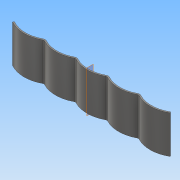
# Autodesk Inventor part: Selection_Selector Sheet
Saved by Autodesk Inventor 2018.1 (Build 221171000, 171)
## iProperties
Created: 2019-02-07
Part Number: Selection_Selector Sheet
Material: Steel, Mild
Document SubType Name: Modeling
Designer: James
Density: 7.85 g/cm^3
Appearance: Semi-Polished
Mass: 244.532 g
Surface Area: 324.289 cm^2
Volume: 31.1506 cm^3
Author: James
Autodesk Inventor part; units mm, degrees
ref_plane "YZ Plane" through (0, 0, 0) normal (1, 0, 0) x (0, 1, 0)
ref_plane "XZ Plane" through (0, 0, 0) normal (0, 1, 0) x (-1, 0, 0)
ref_plane "XY Plane" through (0, 0, 0) normal (0, 0, 1) x (1, 0, 0)
derived "Selection_Skeleton.ipt"
ref_plane "Ground" through (0, 0, 0) normal (0, 1, 0) x (-1, 0, 0)
ref_plane "LHS inner" through (0, 0, 0) normal (1, 0, 0) x (0, 1, 0)
ref_plane "RHS inner" through (300, 0, 0) normal (1, 0, 0) x (0, 1, 0)
ref_plane "Lane 1" through (50, 0, 0) normal (1, 0, 0) x (0, 1, 0)
ref_plane "Lane 2" through (100, 0, 0) normal (1, 0, 0) x (0, 1, 0)
ref_plane "Lane 3" through (150, 0, 0) normal (1, 0, 0) x (0, 1, 0)
ref_plane "Lane 4" through (200, 0, 0) normal (1, 0, 0) x (0, 1, 0)
ref_plane "Lane 5" through (250, 0, 0) normal (1, 0, 0) x (0, 1, 0)
ref_plane "Back" through (0, 0, 0) normal (0, 0, 1) x (1, 0, 0)
sketch "Sketch1" plane through (0, 0, 0) normal (0, 0, 1) x (1, 0, 0)
  line L0 (0, 60) -> (0, -10) projected
  line L1 (300, 60) -> (300, -10) projected
  line L2 (250, 60) -> (250, -10) projected
  line L3 (200, 60) -> (200, -10) projected
  line L4 (150, 60) -> (150, -10) projected
  line L5 (100, 60) -> (100, -10) projected
  line L6 (50, 60) -> (50, -10) projected
  line L7 (-15, 0) -> (90, 0) projected
  arc A0 (25, 9.0244) -> (75, 9.0244) centre (50, 50) ccw
  arc A1 (25, 6.6987) -> (75, 6.6987) centre (50, 50) ccw
  line L8 (25, 9.0244) -> (25, 6.6987)
  line L9 (75, 9.0244) -> (75, 6.6987)
  point P0 (0, 0)
  dimension "d2" = 2
  dimension "d3" = 50
  dimension "d4" = 25
  dimension "d5" = 25
  dimension "d7" = 50
  dimension "d8" = 50
  constraints: 4 end point, 4 point on circle, 2 centre point, 2 vertical alignment, 1 coincident, 1 parallel, 1 point on line, 1 vertical
  measures "d2" radial gap between concentric circles of A0 A1
  measures "d3" distance between parallel lines of L5 L6
  measures "d4" distance from line of L9.start L6
  measures "d5" distance from line of L6 L8.start
  measures "d7" horizontal distance of point (0, 0) A0.centre
  measures "d8" radius of A1
extrude "Extrusion1" add sketch "Sketch1" along normal blind 60
pattern_linear "Rectangular Pattern1" count 5 spacing 50 along (1, 0, 0) of "Extrusion1"
fillet "Fillet1" radius 3 4 edges at (75, 6.6987, 30) (125, 6.6987, 30) (175, 6.6987, 30) (225, 6.6987, 30)
fillet "Fillet2" radius 5 4 edges at (75, 9.0244, 30) (125, 9.0244, 30) (175, 9.0244, 30) (225, 9.0244, 30)
ref_plane "Mid Plane" through (150, 6.6987, 0) normal (-1, 0, 0) x (0, 0, 1)
sketch "Sketch2" plane through (0, 0, 60) normal (0, 0, 1) x (1, 0, 0)
  arc A0 (25, 9.0244) -> (72.6415, 7.6755) centre (50, 50) ccw projected
  arc A1 (25, 6.6987) -> (73.5849, 5.912) centre (50, 50) ccw projected
  line L0 (25, 6.6987) -> (26, 8.4308)
  line L1 (26, 8.4308) -> (50, 50) construction
  line L2 (25, 9.0244) -> (25, 6.6987) projected
  line L3 (25, 6.6987) -> (25, 9.0244)
  line L4 (25, 9.0244) -> (26, 8.4308)
  point P0 (0, 0)
  constraints: 8 end point, 2 collinear, 1 point on circle
extrude "Extrusion2" cut sketch "Sketch2" against normal through all contours A0 L0 L2
mirror "Mirror1" about plane through (150, 6.6987, 0) normal (-1, 0, 0) of "Extrusion2"
equation "\"d4\" = 0.5 * d3"
equation "\"d5\" = d4"
body "Solid1"
